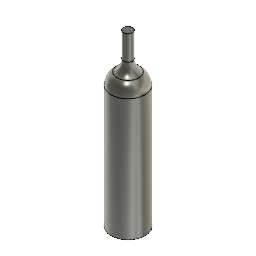
Semana2_Desafio4 (Autodesk Fusion 360 design; units mm, degrees)
Autodesk Fusion 360 part; units mm, degrees
sketch "Sketch1" plane through (0, 0, 0) normal (1, 0, 0) x (0, 1, 0)
  line L0 (0, 0) -> (12.609, 0)
  line L1 (12.609, 0) -> (12.609, 100)
  line L2 (12.609, 100) -> (3.4188, 100)
  line L3 (3.4188, 100) -> (3.4188, 125)
  line L4 (3.4188, 125) -> (0, 125)
  line L5 (0, 125) -> (0, 0)
  constraint coincident L0.start L5.end
  constraint horizontal L0
  constraint perpendicular L0 L1
  constraint perpendicular L1 L2
  constraint perpendicular L2 L3
  constraint perpendicular L1 L4
  constraint perpendicular L0 L5
revolve "Revolve1" add sketch "Sketch1" angle 360 about axis through (0, 0, 125) along (0, 0, -1)
fillet "Fillet3" radius 10 1 edges at (-11.7557, 4.5596, 100)
fillet "Fillet5" radius 10 1 edges at (-3.1874, 1.2363, 100)
